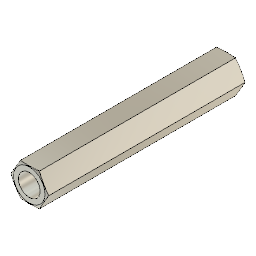
1.500 Standoff (8-32, Aluminum) (Autodesk Fusion 360 design; units mm, degrees)
Autodesk Fusion 360 part; units mm, degrees
sketch "sketch 165" plane through (0, 0, 0) normal (0, 1, 0) x (-1, 0, 0)
  line L0 (3.6662, 0) -> (1.8331, 3.175)
  line L1 (0, 3.175) -> (-1.8331, 3.175)
  line L2 (-1.8331, 3.175) -> (-3.6662, 0)
  line L3 (-3.6662, 0) -> (-1.8331, -3.175)
  line L4 (-1.8331, -3.175) -> (0, -3.175)
  line L5 (0, -3.175) -> (1.8331, -3.175)
  line L6 (1.8331, -3.175) -> (3.6662, 0)
  line L7 (3.6662, 0) -> (1.8331, 3.175)
  line L8 (1.8331, 3.175) -> (0, 3.175)
  circle A0 centre (0, 0) radius 2.0955
extrude "Extrude1" add sketch "sketch 165" along normal blind 38.1 contours L0 L1 L2 L3 L4 L5 L6 L7 L8 | A0
extrude "Extrude2" cut sketch "sketch 165" along normal blind 12.7 contours A0
extrude "Extrude3" cut sketch "sketch 165" against normal blind 12.7 from surface at 38.1 contours A0
ref_plane "WorkPlane1" through (19.05, 0, 0) normal (1, 0, 0) x (0, 1, 0)
sketch "Sketch1" plane through (0, 0, 0) normal (1, 0, 0) x (0, 1, 0)
  arc A0 (0, -3.0312) -> (0.127, -3.6662) centre (1.651, -3.0312) ccw
  line L0 (0.127, -3.6662) -> (0, -3.6662)
  line L1 (0, -3.6662) -> (0, -3.0312)
  line L2 (0, 0) -> (0, -3.0312) construction
  line L3 (19.05, -3.175) -> (19.05, 3.175) construction
  line L4 (38.1, -3.6662) -> (38.1, -3.0312)
  line L5 (37.973, -3.6662) -> (38.1, -3.6662)
  arc A1 (37.973, -3.6662) -> (38.1, -3.0312) centre (36.449, -3.0312) ccw
  line L6 (0, 0) -> (19.05, 0) construction
  dimension "d8" = 1.651
  dimension "d9" = 0.635
  dimension "d11" = 3.0312
  dimension "d13" = 19.05
  dimension "d14" = 6.35
  constraint horizontal L0
  constraint tangent A0 L1
  constraint coincident L2.start L6.start
  constraint tangent A0 L2
  constraint vertical L2
  constraint vertical L3
  constraint symmetric A0.end L3 L5.start
  constraint symmetric A0.start L3 L4.end
  constraint symmetric A0 L3 A1
  constraint symmetric L0.end L3 L4.start
  constraint midpoint L3 L6.end
  constraint horizontal L6
  measures "d8" radius of A0
  measures "d9" vertical distance of A0.end A0.start
  measures "d11" distance of L2.start A0.start
  measures "d13" distance of L2.start L3
  measures "d14" distance of L3.start L3.end
revolve "Revolve1" cut sketch "Sketch1" angle 360 about axis through (0, 0, 0) along (0, 1, 0)
equation "length_distance = 1.500 in"
equation "d3 = min(length_distance / 2; 0.5 in)"
equation "d6 = -min(length_distance / 2; 0.5 in)"
equation "d12 = length_distance / 2"
equation "d13 = length_distance / 2"
